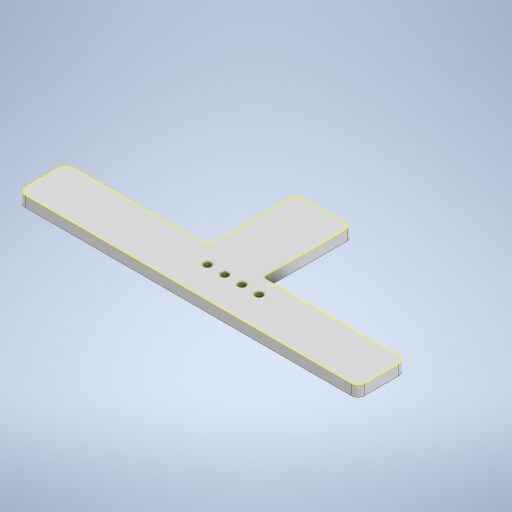
# Autodesk Inventor part: pcb_dolne
Saved by Autodesk Inventor 2023 (Build 270158000, 158)
## iProperties
Created: 2023-12-23
Part Number: pcb_dolne
Material: Ogólny
Document SubType Name: Modeling
Designer: Kamil
Density: 1 g/cm^3
Appearance: Domyślna
Author: Kamil
Autodesk Inventor part; units mm, degrees
ref_plane "YZ Plane" through (0, 0, 0) normal (1, 0, 0) x (0, 1, 0)
ref_plane "XZ Plane" through (0, 0, 0) normal (0, 1, 0) x (-1, 0, 0)
ref_plane "XY Plane" through (0, 0, 0) normal (0, 0, 1) x (1, 0, 0)
sketch "Szkic1" plane through (0, 0, 0) normal (0, 1, 0) x (-1, 0, 0)
  line L0 (0, 0) -> (50, 0)
  line L1 (50, 0) -> (50, -7)
  line L2 (50, -7) -> (0, -7)
  line L3 (0, -7) -> (0, 0)
  dimension "d0" = 50
  dimension "d1" = 7
  constraints: 8 end point, 2 parallel, 1 horizontal, 1 perpendicular
  measures "d0" distance of L1.end L2.end
  measures "d1" distance of L0.end L1.end
extrude "Wyciągnięcie proste1" add sketch "Szkic1" along normal blind 1.6
fillet "Zaokrąglenie1" radius 1 4 edges at (0, 0.8, 0) (0, 0.8, -7) (-50, 0.8, 0) (-50, 0.8, -7)
sketch "Szkic2" plane through (0, 0, 0) normal (0, -1, 0) x (1, 0, 0)
  line L0 (-1, -7) -> (-49, -7) projected
  line L1 (-30, -19.9397) -> (-30, -7.5897) projected
  line L2 (-20, -7.5897) -> (-20, -19.9397) projected
  line L3 (-20, -7) -> (-30, -7)
  line L4 (-30, -7) -> (-30, -21)
  line L5 (-30, -21) -> (-20, -21)
  line L6 (-20, -21) -> (-20, -7)
  line L7 (-21, -20) -> (-29, -20)
  line L8 (-29, -20) -> (-29, -8)
  line L9 (-29, -8) -> (-21, -8)
  line L10 (-21, -8) -> (-21, -20)
  line L11 (-1, -7) -> (-49, -7) projected
  line L12 (-29, -8) -> (-21, -8)
  line L13 (-21, -8) -> (-21, -7)
  line L14 (-21, -7) -> (-29, -7)
  line L15 (-29, -7) -> (-29, -8)
  point P0 (0, 0)
  dimension "d5" = 14
  constraints: 24 end point, 6 parallel, 3 perpendicular, 3 point on line, 2 horizontal, 3 other
  measures "d5" distance of L4.end L3.end
extrude "Wyciągnięcie proste2" add sketch "Szkic2" against normal up to surface (1.6 mm away) contours L13 L9 L15 L0 | L10 L7 L8 L9
sketch "Szkic3" plane through (0, 1.6, 0) normal (0, 1, 0) x (1, 0, 0)
  line L0 (-28.2, 1.9426) -> (-28.2, 7.0897) projected
  line L1 (-17.5, 7.0897) -> (-17.5, 1.9426) projected
  line L2 (-28.2, 4.5162) -> (-17.5, 4.5162) construction
  circle A0 centre (-26.66, 4.5162) radius 0.55
  circle A1 centre (-24.12, 4.5162) radius 0.55
  circle A2 centre (-21.58, 4.5162) radius 0.55
  circle A3 centre (-19.04, 4.5162) radius 0.55
  point P0 (0, 0)
  dimension "d9" = 1.1
  dimension "d12" = 2.54
  dimension "d17" = 1.54
  constraints: 4 centre point, 2 end point, 2 midpoint, 1 horizontal, 1 point on line, 6 other
  measures "d9" diameter of A0
  measures "d12" distance of A0.centre A1.centre
  measures "d17" distance from line of A0.centre L0
extrude "Wyciągnięcie proste3" cut sketch "Szkic3" against normal through all
fillet "Zaokrąglenie3" radius 0.5 4 edges at (-21, 0.8, -20) (-29, 0.8, -20) (-29, 0.8, -7) (-21, 0.8, -7)
sketch "Szkic6" plane through (0, 1.6, 0) normal (0, 1, 0) x (1, 0, 0)
  point P0 (0, 0)
sketch "Szkic7" plane through (0, 1.6, 0) normal (0, 1, 0) x (1, 0, 0)
  arc A0 (-28.5, 20) -> (-29, 19.5) centre (-28.5, 19.5) ccw projected
  line L0 (-29, 7.5) -> (-29, 19.5) projected
  arc A1 (-29.5, 7) -> (-29, 7.5) centre (-29.5, 7.5) ccw projected
  line L1 (-29.5, 7) -> (-49, 7) projected
  arc A2 (-49, 7) -> (-50, 6) centre (-49, 6) ccw projected
  line L2 (-50, 6) -> (-50, 1) projected
  arc A3 (-50, 1) -> (-49, 0) centre (-49, 1) ccw projected
  line L3 (-49, 0) -> (-1, 0) projected
  arc A4 (-1, 0) -> (0, 1) centre (-1, 1) ccw projected
  line L4 (0, 1) -> (0, 6) projected
  arc A5 (0, 6) -> (-1, 7) centre (-1, 6) ccw projected
  line L5 (-1, 7) -> (-20.5, 7) projected
  arc A6 (-21, 7.5) -> (-20.5, 7) centre (-20.5, 7.5) ccw projected
  line L6 (-21, 19.5) -> (-21, 7.5) projected
  arc A7 (-21, 19.5) -> (-21.5, 20) centre (-21.5, 19.5) ccw projected
  line L7 (-28.5, 20) -> (-21.5, 20) projected
  circle A8 centre (-21.58, 4.5162) radius 0.55 projected
  circle A9 centre (-24.12, 4.5162) radius 0.55 projected
  circle A10 centre (-19.04, 4.5162) radius 0.55 projected
  circle A11 centre (-26.66, 4.5162) radius 0.55 projected
  point P0 (0, 0)
